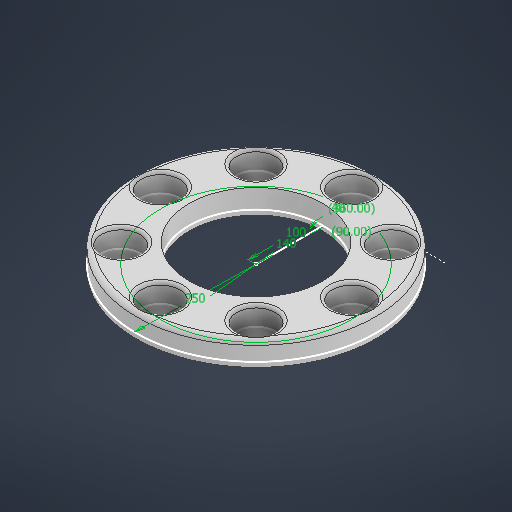
# Autodesk Inventor part: Baseplate
Saved by Autodesk Inventor 2026.2 (Build 302298000, 298)
## iProperties
Created: 2026-03-16
Part Number: Baseplate
Material: Generic
Document SubType Name: Modeling
Designer: Cobble
Density: 1 g/cm^3
Appearance: Default
Author: Cobble
Autodesk Inventor part; units mm, degrees
ref_plane "YZ Plane" through (0, 0, 0) normal (1, 0, 0) x (0, 1, 0)
ref_plane "XZ Plane" through (0, 0, 0) normal (0, 1, 0) x (-1, 0, 0)
ref_plane "XY Plane" through (0, 0, 0) normal (0, 0, 1) x (1, 0, 0)
sketch "Sketch1" plane through (0, 0, 0) normal (0, 0, 1) x (1, 0, 0)
  circle A0 centre (0, 0) radius 20
  line L0 (0, 0) -> (0, -100)
  line L1 (0, 0) -> (100, 0) construction
  circle A1 centre (-70.7107, -29.2893) radius 20
  circle A2 centre (-100, -100) radius 20
  circle A3 centre (-70.7107, -170.7107) radius 20
  circle A4 centre (0, -200) radius 20
  circle A5 centre (70.7107, -170.7107) radius 20
  circle A6 centre (100, -100) radius 20
  circle A7 centre (70.7107, -29.2893) radius 20
  circle A8 centre (0, -100) radius 125
  circle A9 centre (0, -100) radius 70
  dimension "d0" = 40
  dimension "d1" = 100
  dimension "d2" = 90
  dimension "d5" = 360
  dimension "d7" = 250
  dimension "d9" = 140
  constraints: 10 centre point, 4 end point, 3 coincident, 1 horizontal, 1 perpendicular, 1 vertical, 17 other
  measures "d0" diameter of A0
  measures "d1" distance of L0.start L0.end
  measures "d2" angle of L0 L1
  measures "d7" diameter of A8
  measures "d9" diameter of A9
extrude "Extrusion1" add sketch "Sketch1" along normal blind 20
extrude "Extrusion2" add sketch "Sketch1" against normal blind 5 contours A0 | A1 | A2 | A3 | A4 | A5 | A6 | A7 | A8
fillet "Fillet1" radius 3 8 edges at (-90.7107, -170.7107, 20) (-120, -100, 20) (-90.7107, -29.2893, 20) (-20, 0, 20) (50.7107, -29.2893, 20) (80, -100, 20) (50.7107, -170.7107, 20) (-20, -200, 20)
fillet "Fillet2" radius 5 1 edges at (-125, -100, 20)
body "Solid1"
